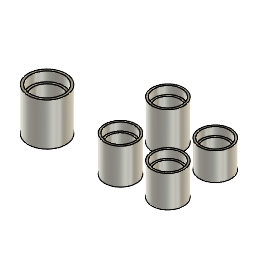
20251012_Laser_Lens_Standoff (Autodesk Fusion 360 design; units mm, degrees)
part number: 2025-10-15-01-45-27-477
Autodesk Fusion 360 part; units mm, degrees
sketch "Sketch1" plane through (0, 0, 0) normal (0, 0, 1) x (1, 0, 0)
  circle A0 centre (10, 10) radius 4
  circle A1 centre (10, 10) radius 2.1
  circle A2 centre (10, 10) radius 2.1
  circle A3 centre (10, 10) radius 4
  circle A4 centre (22, 10) radius 2.1
  circle A5 centre (22, 10) radius 4
  circle A6 centre (22, 10) radius 4
  circle A7 centre (22, 10) radius 2.1
  circle A8 centre (22, -2) radius 4
  circle A9 centre (22, -2) radius 2.1
  circle A10 centre (22, -2) radius 2.1
  circle A11 centre (22, -2) radius 4
  circle A12 centre (22, -2) radius 4
  circle A13 centre (22, -2) radius 2.1
  circle A14 centre (22, -2) radius 2.1
  circle A15 centre (22, -2) radius 4
  circle A16 centre (9, -2) radius 4
  circle A17 centre (9, -2) radius 2.1
  circle A18 centre (9, -2) radius 2.1
  circle A19 centre (9, -2) radius 4
  circle A20 centre (9, -2) radius 4
  circle A21 centre (9, -2) radius 4
  circle A22 centre (9, -2) radius 2.1
  circle A23 centre (9, -2) radius 2.1
  dimension "d1" = 8
  dimension "d2" = 4.2
  dimension "d3" = 8
  dimension "d4" = 4.2
  dimension "d5" = 8
  dimension "d6" = 4.2
  dimension "d7" = 8
  dimension "d8" = 4.2
  dimension "d9" = 8
  dimension "d10" = 4.2
  dimension "d11" = 8
  dimension "d12" = 4.2
  dimension "d13" = 8
  dimension "d14" = 4.2
  dimension "d15" = 8
  dimension "d16" = 4.2
  dimension "d17" = 8
  dimension "d18" = 4.2
  dimension "d19" = 8
  dimension "d20" = 4.2
  dimension "d21" = 8
  dimension "d22" = 4.2
  dimension "d23" = 8
  dimension "d24" = 4.2
  constraint concentric A0 A1
  constraint concentric A2 A3
  constraint concentric A5 A7
  constraint concentric A4 A6
  constraint concentric A10 A11
  constraint concentric A8 A9
  constraint concentric A13 A15
  constraint concentric A12 A14
  constraint concentric A21 A22
  constraint concentric A16 A18
  constraint concentric A17 A20
  constraint concentric A19 A23
  measures "d1" diameter of A0
  measures "d2" diameter of A1
  measures "d3" diameter of A3
  measures "d4" diameter of A2
  measures "d5" diameter of A5
  measures "d6" diameter of A7
  measures "d7" diameter of A6
  measures "d8" diameter of A4
  measures "d9" diameter of A11
  measures "d10" diameter of A10
  measures "d11" diameter of A8
  measures "d12" diameter of A9
  measures "d13" diameter of A15
  measures "d14" diameter of A13
  measures "d15" diameter of A12
  measures "d16" diameter of A14
  measures "d17" diameter of A21
  measures "d18" diameter of A22
  measures "d19" diameter of A16
  measures "d20" diameter of A18
  measures "d21" diameter of A20
  measures "d22" diameter of A17
  measures "d23" diameter of A19
  measures "d24" diameter of A23
extrude "Extrude1" add sketch "Sketch1" along normal blind 2 contours A16 A19 A20 A21 makes body 1
sketch "Sketch2" plane through (0, 0, 2) normal (0, 0, 1) x (-1, 0, 0)
  circle A0 centre (-9, 2) radius 2.1
  circle A1 centre (-9, 2) radius 4
  circle A2 centre (-9, 2) radius 2.1
  circle A3 centre (-9, 2) radius 4
  circle A4 centre (-9, 2) radius 3
  dimension "d27" = 6
  constraint concentric A2 A4
  measures "d27" diameter of A4
extrude "Extrude2" add sketch "Sketch2" along normal blind 3 contours A1 A3 bodies 1
copy_body "CopyPasteBodies1" bodies 1 makes body 2
move_body "Move1" bodies 2 to x (1, 0, 0) y (0, 1, 0) z (0, 0, 1) at (0, -12, 0)
copy_body "CopyPasteBodies2" bodies 1 makes body 3
move_body "Move2" bodies 3 to x (1, 0, 0) y (0, 1, 0) z (0, 0, 1) at (-12, 0, 0)
copy_body "CopyPasteBodies3" bodies 1 makes body 4
move_body "Move3" bodies 4 to x (1, 0, 0) y (0, 1, 0) z (0, 0, 1) at (-11, -13, 0)
extrude "Extrude3" add 1 faces at (5.3482, -13.8013, 5) along direction (0, 0, 1) blind 1 on bodies 2 bodies 2
extrude "Extrude4" add 1 faces at (-5.6406, -14.6522, 5) along direction (0, 0, 1) blind 2 on bodies 4 bodies 4
extrude "Extrude5" add 1 faces at (-6.6406, -1.6522, 5) along direction (0, 0, 1) blind 3 on bodies 3 bodies 3
sketch "Sketch3" plane through (0, 0, 5) normal (0, 0, 1) x (-1, 0, 0)
  circle A0 centre (-9, 2) radius 3
  circle A1 centre (-9, 2) radius 4
  circle A2 centre (-9, 2) radius 3.5
  dimension "d36" = 7
  constraint concentric A0 A2
  measures "d36" diameter of A2
extrude "Extrude6" add sketch "Sketch3" along normal blind 2 contours A1 bodies 1
sketch "Sketch4" plane through (0, 0, 8) normal (0, 0, 1) x (-1, 0, 0)
  circle A0 centre (3, 2) radius 3
  circle A1 centre (3, 2) radius 4
  circle A2 centre (3, 2) radius 3.5
  dimension "d39" = 7
  constraint concentric A0 A2
  measures "d39" diameter of A2
extrude "Extrude7" add sketch "Sketch4" along normal blind 2 contours A1 bodies 3
sketch "Sketch5" plane through (0, 0, 7) normal (0, 0, 1) x (-1, 0, 0)
  circle A0 centre (2, 15) radius 3
  circle A1 centre (2, 15) radius 4
  circle A2 centre (2, 15) radius 3.5
  dimension "d42" = 7
  constraint concentric A0 A2
  measures "d42" diameter of A2
extrude "Extrude8" add sketch "Sketch5" along normal blind 2 contours A1 bodies 4
sketch "Sketch6" plane through (0, 0, 6) normal (0, 0, 1) x (-1, 0, 0)
  circle A0 centre (-9, 14) radius 3
  circle A1 centre (-9, 14) radius 4
  circle A2 centre (-9, 14) radius 3.5
  dimension "d45" = 7
  constraint concentric A0 A2
  measures "d45" diameter of A2
extrude "Extrude9" add sketch "Sketch6" along normal blind 2 contours A1 bodies 2
sketch "Sketch7" plane through (0, 0, 0) normal (0, 0, 1) x (1, 0, 0)
copy_body "CopyPasteBodies4" bodies 2 makes body 5
copy_body "CopyPasteBodies5" bodies 4 makes body 6
move_body "Move4" bodies 6 to x (1, 0, 0) y (0, 1, 0) z (0, 0, 1) at (-18, 0, 0)
scale "Scale1" factor 1.2 about (-17, -15, 2) bodies 6
